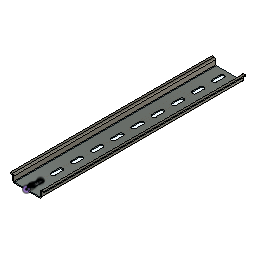
2x-lrs-psu (Autodesk Fusion 360 archive; units mm, degrees)
design "Cheap Aluminium DIN Rail [Parametric]"
Autodesk Fusion 360 part; units mm, degrees
sketch "Skizze1" plane through (0, 0, 0) normal (0, 1, 0) x (1, 0, 0)
  line L0 (14.5, -1) -> (-13.5, -1)
  line L1 (-13.5, -1) -> (-13.5, 0)
  line L2 (-13.5, 0) -> (14.5, 0)
  line L3 (14.5, 0) -> (14.5, -1)
  line L4 (14.5, -1) -> (-13.5, 0) construction
  line L5 (-13.5, -1) -> (14.5, 0) construction
  line L6 (-13.5, 0) -> (-12.5, 0)
  line L7 (-12.5, 0) -> (-12.5, -7.5)
  line L8 (-12.5, -7.5) -> (-13.5, -7.5)
  line L9 (-13.5, -7.5) -> (-13.5, 0)
  line L10 (14.5, 0) -> (13.5, 0)
  line L11 (13.5, 0) -> (13.5, -7.5)
  line L12 (13.5, -7.5) -> (14.5, -7.5)
  line L13 (14.5, -7.5) -> (14.5, 0)
  line L14 (-12.5, -7.5) -> (-16.15, -7.5)
  line L15 (-16.15, -7.5) -> (-16.15, -6.5)
  line L16 (-16.15, -6.5) -> (-12.5, -6.5)
  line L17 (-12.5, -6.5) -> (-12.5, -7.5)
  line L18 (13.5, -7.5) -> (17.15, -7.5)
  line L19 (17.15, -7.5) -> (17.15, -6.5)
  line L20 (17.15, -6.5) -> (13.5, -6.5)
  line L21 (13.5, -6.5) -> (13.5, -7.5)
  point P0 (0.5, -0.5)
  dimension "d7" = 28
  dimension "d8" = 1
  dimension "d9" = 7.5
  dimension "d10" = 1
  dimension "d11" = 7.5
  dimension "d12" = 1
  dimension "d13" = 3.65
  dimension "d14" = 1
  dimension "d15" = 3.65
  dimension "d16" = 1
  constraint perpendicular L0 L1
  constraint parallel L0 L2
  constraint parallel L1 L3
  constraint horizontal L0
  constraint coincident L4 P0
  constraint coincident L5 P0
  constraint horizontal L6
  constraint vertical L7
  constraint horizontal L8
  constraint vertical L9
  constraint horizontal L10
  constraint vertical L11
  constraint horizontal L12
  constraint vertical L13
  constraint horizontal L14
  constraint vertical L15
  constraint horizontal L16
  constraint vertical L17
  constraint horizontal L18
  constraint vertical L19
  constraint horizontal L20
  constraint vertical L21
  measures "d7" distance of L1.end L2.end
  measures "d8" distance of L0.end L1.end
  measures "d9" distance of L1.end L8.end
  measures "d10" distance of L1.end L6.end
  measures "d11" distance of L2.end L12.end
  measures "d12" distance of L2.end L10.end
  measures "d13" distance of L7.end L14.end
  measures "d14" distance of L7.end L16.end
  measures "d15" distance of L11.end L18.end
  measures "d16" distance of L11.end L20.end
extrude "Extrusion1" add sketch "Skizze1" along normal blind 200
fillet "Abrundung1" radius 1.5 4 edges at (13.5, 100, 7.5) (-12.5, 100, 7.5) (14.5, 100, 0) (-13.5, 100, 0)
fillet "Abrundung2" radius 0.5 4 edges at (-13.5, 100, 6.5) (14.5, 100, 6.5) (13.5, 100, 1) (-12.5, 100, 1)
sketch "Skizze2" plane through (0, 0, 1) normal (0, 0, 1) x (-1, 0, 0)
  line L0 (12, -200) -> (12, 0)
  line L1 (12, 0) -> (-13, 0)
  line L2 (-13, 0) -> (-13, -200)
  line L3 (-13, -200) -> (12, -200)
  line L4 (0, 0) -> (0, -4.15) construction
  line L5 (-2.05, -6.2) -> (-2.05, -13.8)
  arc A0 (-2.05, -13.8) -> (2.05, -13.8) centre (0, -13.8) ccw
  line L6 (2.05, -13.8) -> (2.05, -6.2)
  arc A1 (2.05, -6.2) -> (-2.05, -6.2) centre (0, -6.2) ccw
  line L7 (0, -4.15) -> (0, -15.85) construction
  point P0 (0, -4.15)
  dimension "d26" = 4.15
  dimension "d34" = 11.7
  dimension "d35" = 4.1
  constraint coincident L4.start origin
  constraint perpendicular L3 L4
  constraint coincident P0 L4.end
  constraint tangent L5 A0
  constraint tangent A0 L6
  constraint parallel L5 L6
  constraint tangent L6 A1
  constraint tangent L5 A1
  constraint midpoint P0 A1
  constraint midpoint A0 L7.end
  constraint parallel L4 L7
  measures "d26" distance of L4.start P0
  measures "d34" distance of P0 L7.end
  measures "d35" diameter of A0
extrude "Extrusion2" cut sketch "Skizze2" against normal blind 1 contours L5 A0 L6 A1
pattern_linear "R-Anordnung1" count 10 spacing 20 along (0, 1, 0) of "Extrusion2"
equation "InnerWidth = 28 mm" comment "BI"
equation "OuterWidth = 35.3 mm" comment "35"
equation "Height = 7.5 mm" comment "h"
equation "Thickness = 1 mm" comment "D"
equation "Length = 200 mm" comment "L"
equation "SlotDistance = 25 mm" comment "ALL"
equation "d7 = InnerWidth"
equation "d8 = Thickness"
equation "d9 = Height"
equation "d10 = Thickness"
equation "d11 = Height"
equation "d12 = Thickness"
equation "d13 = ( OuterWidth - InnerWidth ) / 2"
equation "d14 = Thickness"
equation "d15 = ( OuterWidth - InnerWidth ) / 2"
equation "d16 = Thickness"
equation "d17 = Length"
equation "OuterFillet = 1.5 mm" comment "R"
equation "d20 = OuterFillet"
equation "InnerFillet = OuterFillet - Thickness" comment "RK"
equation "d22 = InnerFillet"
equation "SlotWidth = 4.1 mm" comment "LLB"
equation "SlotLength = 11.7 mm" comment "LLH"
equation "SlotDistance2 = 20 mm" comment "LLA"
equation "d26 = ( ( Length - ( ( Length / SlotDistance2 ) * SlotLength ) ) / ( Length / SlotDistance2 ) ) / 2"
equation "d28 = -Thickness"
equation "d30 = Length / SlotDistance2"
equation "d32 = SlotDistance2"
equation "d34 = SlotLength"
equation "d35 = SlotWidth"
